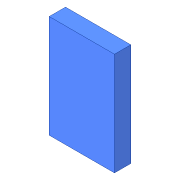
# Autodesk Inventor part: 2479 Adafruit Bluefruit LE UART Friend
Saved by Autodesk Inventor 2018.3 (Build 223284000, 284)
## iProperties
Created: 2018-12-11
Part Number: 2479 Adafruit Bluefruit LE UART Friend
Material: Generic
Document SubType Name: Modeling
Designer: tei06398
Mass: 3.30363 g
Surface Area: 18.3225 cm^2
Volume: 3.30363 cm^3
Density: 1 g/cm^3
Appearance: Default
Author: tei06398
Autodesk Inventor part; units mm, degrees
ref_plane "YZ Plane" through (0, 0, 0) normal (1, 0, 0) x (0, 1, 0)
ref_plane "XZ Plane" through (0, 0, 0) normal (0, 1, 0) x (-1, 0, 0)
ref_plane "XY Plane" through (0, 0, 0) normal (0, 0, 1) x (1, 0, 0)
sketch "Sketch1" plane through (0, 0, 0) normal (0, 0, 1) x (1, 0, 0)
  line L0 (0, 0) -> (20.32, 0)
  line L1 (20.32, 0) -> (20.32, 32.004)
  line L2 (20.32, 32.004) -> (0, 32.004)
  line L3 (0, 32.004) -> (0, 0)
  dimension "d0" = 20.32
  dimension "d1" = 32.004
  constraints: 8 end point, 2 parallel, 1 horizontal, 1 perpendicular
  measures "d0" distance of L2.end L1.end
  measures "d1" distance of L1.end L0.end
extrude "Extrusion1" add sketch "Sketch1" against normal blind 5.08
body "Solid1"
